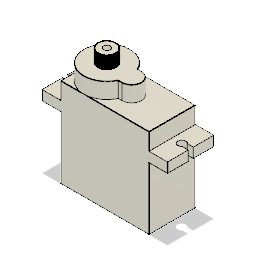
_Servo 2.321842c1-610b-42d5-ac31-599ccc053177_LV0 (Autodesk Fusion 360 design; units mm, degrees)
Autodesk Fusion 360 part; units mm, degrees
note: some values were not read from the file. Set by a fixed rule: which sketch regions a step uses.
sketch "Sketch1" plane through (0, 0, 0) normal (0, 0, 1) x (1, 0, 0)
  line L0 (0, 0) -> (0, 4.3)
  line L1 (0, -18.4) -> (0, -2.5)
  line L2 (0, -2.5) -> (-4.7, -2.5)
  line L3 (-4.7, -2.5) -> (-4.7, 0)
  line L4 (-4.7, 0) -> (0, 0)
  line L5 (22.5, 0) -> (22.5, 4.3)
  line L6 (27.2, 0) -> (22.5, 0)
  line L7 (27.2, -2.5) -> (27.2, 0)
  line L8 (22.5, -2.5) -> (27.2, -2.5)
  line L9 (22.5, -18.4) -> (22.5, -2.5)
  line L10 (0, -18.4) -> (22.5, -18.4)
  line L11 (0, 4.3) -> (22.5, 4.3)
  dimension "d2" = 4.7
  dimension "d3" = 2.5
  dimension "d4" = 15.9
  dimension "d5" = 22.7
  dimension "d7" = 22.5
  dimension "d9" = 22.5
  dimension "d10" = 15.9
  constraint coincident L0.start L4.end
  constraint vertical L0
  constraint perpendicular L1 L2
  constraint perpendicular L2 L3
  constraint perpendicular L0 L4
  constraint perpendicular L9 L10
  constraint perpendicular L5 L11
  constraint parallel L1 L9
  constraint parallel L0 L5
  constraint parallel L6 L8
  constraint parallel L2 L4
  measures "d2" distance of L3.end L0.start
  measures "d3" distance of L2.end L3.end
  measures "d4" distance of L1.start L1.end
  measures "d5" distance of L0.end L1.start
  measures "d7" distance of L0.end L5.end
  measures "d9" distance of L1.start L9.start
  measures "d10" distance of L8.start L9.start
extrude "Extrude1" add sketch "Sketch1" along normal blind 11.8 contours L0 L1 L2 L3 L4 L5 L6 L7 L8 L9 L10 L11 picked at (7.5, -7.8) makes body 1
sketch "Sketch6" plane through (0, 4.3, 0) normal (0, 1, 0) x (-1, 0, 0)
  line L0 (-22.5, 0) -> (0, 0)
  line L1 (0, 0) -> (0, 11.8)
  line L2 (0, 11.8) -> (-22.5, 11.8)
  line L3 (-22.5, 11.8) -> (-22.5, 0)
  line L4 (-11.244156, 3.4) -> (-12.2, 3.4)
  arc A0 (-12.2, 8.4) -> (-12.2, 3.4) centre (-12.2, 5.9) ccw
  line L5 (-12.2, 8.4) -> (-11.244156, 8.4)
  arc A1 (-11.244156, 3.4) -> (-11.244156, 8.4) centre (-5.9, 5.9) ccw
  dimension "d69" = 11.8
  dimension "d71" = 5
  dimension "d72" = 3.4
  dimension "d73" = 10.3
  constraint tangent L0 A1
  constraint tangent L1 A1
  constraint parallel L2 L4
  constraint tangent L4 A0
  constraint tangent A0 L5
  constraint parallel L4 L5
  measures "d69" diameter of A1
  measures "d71" distance of L4 L5
  measures "d72" distance of L0 L4
  measures "d73" distance of L3 A0.centre
extrude "Extrude9" add sketch "Sketch6" along normal blind 4 contours L4 A0 L5 A1 picked at (-7.380628, 5.376962) bodies 1
sketch "Sketch7" plane through (0, 8.3, 0) normal (0, 1, 0) x (-1, 0, 0)
  arc A0 (-12.2, 8.4) -> (-12.2, 3.4) centre (-12.2, 5.9) ccw
  line L0 (-12.2, 3.4) -> (-11.244156, 3.4)
  arc A1 (-11.244156, 3.4) -> (-11.244156, 8.4) centre (-5.9, 5.9) ccw
  line L1 (-11.244156, 8.4) -> (-12.2, 8.4)
  circle A2 centre (-5.9, 5.9) radius 2.3
  line L2 (-5.9, 11.8) -> (0, 11.8)
  dimension "d77" = 4.6
  constraint concentric A1 A2
  measures "d77" diameter of A2
extrude "Extrude10" add sketch "Sketch7" along normal blind 3.2 separate body contours A2 picked at (-7.201969, 6.065119) makes body 2
sketch "Sketch8" plane through (0, 11.5, 0) normal (0, 1, 0) x (-1, 0, 0)
  circle A0 centre (-5.9, 5.9) radius 2.3
  circle A1 centre (-5.9, 5.9) radius 0.85
  line L0 (-5.927716, 8.066913) -> (-6, 8.241421)
  line L1 (-6, 8.241421) -> (-5.8, 8.241421)
  line L2 (-5.8, 8.241421) -> (-5.872284, 8.066913)
  arc A2 (-5.927716, 8.066913) -> (-5.872284, 8.066913) centre (-5.9, 8.078394) ccw
  point P0 (-5.9, 8)
  dimension "d81" = 1.7
  dimension "d84" = 0.1
  dimension "d85" = 0.1
  dimension "d86" = 45
  dimension "d88" = 2.1
  dimension "d94" = 0.03
  constraint concentric A0 A1
  constraint coincident P0 L0
  constraint coincident P0 L2
  constraint tangent L0 A2
  constraint tangent L2 A2
  measures "d81" diameter of A1
  measures "d86" angle of L0 L2
  measures "d88" distance of A0.centre P0
  measures "d94" radius of A2
extrude "Extrude11" cut sketch "Sketch8" against normal blind 3.2 contours A1 picked at (-6.010624, 5.693552) bodies 2
extrude "Extrude12" cut sketch "Sketch8" against normal blind 3.2 contours A0 L0 L2 A2 | A0 L0 L1 L2 picked at (-5.909139, 8.111221) picked at (-5.909139, 8.22756) bodies 2
fillet "Fillet4" radius 0.01 2 edges at (5.817766, 9.9, 8.198529) (5.982234, 9.9, 8.198529) on bodies 2
pattern_circular "C-Pattern2" count 80 over 360 about axis through (5.9, 11.5, 5.9) along (0, 1, 0) of "Extrude12", "Fillet4"
sketch "Sketch9" plane through (0, 0, 0) normal (0, 1, 0) x (-1, 0, 0)
  line L0 (0, 0) -> (4.7, 0)
  line L1 (4.7, 0) -> (4.7, 11.8)
  line L2 (4.7, 11.8) -> (0, 11.8)
  line L3 (0, 11.8) -> (0, 0)
  line L4 (3, 5.25) -> (4.7, 5.25)
  line L5 (3, 6.55) -> (4.7, 6.55)
  arc A0 (3.159934, 6.55) -> (3.159934, 5.25) centre (2.4, 5.9) ccw
  line L6 (-27.2, 0) -> (-27.2, 11.8)
  line L7 (-27.2, 11.8) -> (-22.5, 11.8)
  line L8 (-27.2, 6.55) -> (-25.5, 6.55)
  line L9 (-27.2, 5.25) -> (-25.5, 5.25)
  arc A1 (-25.659934, 5.25) -> (-25.659934, 6.55) centre (-24.9, 5.9) ccw
  dimension "d95" = 2
  dimension "d96" = 2.3
  dimension "d97" = 1.3
  dimension "d99" = 5.9
  dimension "d100" = 0.65
  dimension "d101" = 2
  dimension "d102" = 2.3
  dimension "d103" = 5.9
  dimension "d104" = 1.3
  dimension "d105" = 0.65
  constraint coincident L1 L4.end
  constraint perpendicular L1 L4
  constraint coincident L1 L5.end
  constraint perpendicular L1 L5
  constraint coincident L6 L8.start
  constraint perpendicular L6 L8
  constraint coincident L6 L9.start
  constraint perpendicular L6 L9
  measures "d95" diameter of A0
  measures "d96" distance of L1 A0.centre
  measures "d97" distance of L4 L5
  measures "d99" distance of L2 A0.centre
  measures "d100" distance of A0.centre L5
  measures "d101" diameter of A1
  measures "d102" distance of A1.centre L6
  measures "d103" distance of A1.centre L7
  measures "d104" distance of L8 L9
  measures "d105" distance of A1.centre L8
extrude "Extrude13" cut sketch "Sketch9" against normal through all contours L1 L4 L5 A0 | L6 L8 L9 A1 picked at (3.673289, 5.683333) picked at (-25.074196, 5.924564) bodies 1
fillet "Fillet5" radius 0.1 27 edges at (0, 8.3, 5.9) (11.722078, 8.3, 8.4) (14.7, 8.3, 5.9) (11.722078, 8.3, 3.4) (14.2, 4.3, 11.8) (22.5, 4.3, 5.9) (14.2, 4.3, 0) (2.95, 4.3, 11.8) (0, 4.3, 8.85) (0, 4.3, 2.95) (2.95, 4.3, 0) (-4.7, -1.25, 11.8) (11.25, -18.4, 11.8) (0, -18.4, 5.9) (11.25, -18.4, 0) (22.5, -18.4, 5.9) (22.5, -10.45, 0) (22.5, -10.45, 11.8) (27.2, -1.25, 11.8) (27.2, -1.25, 0) (22.5, 2.15, 11.8) (22.5, 2.15, 0) (0, -10.45, 0) (-4.7, -1.25, 0) (0, 2.15, 0) (0, 2.15, 11.8) (0, -10.45, 11.8) on bodies 1
combine "Combine1" operation add target body 2 tool bodies 1
equation "d85 = d84"
